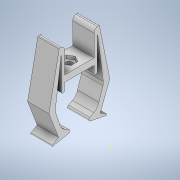
# Autodesk Inventor part: защёлка_выдача2
Saved by Autodesk Inventor 2020 (Build 240168000, 168)
## iProperties
Created: 2022-07-29
Part Number: защёлка_выдача2
Material: Типовые
Document SubType Name: Modeling
Designer: akapu
Density: 1 g/cm^3
Appearance: По умолчанию
Author: akapu
Autodesk Inventor part; units mm, degrees
ref_plane "YZ Plane" through (0, 0, 0) normal (1, 0, 0) x (0, 1, 0)
ref_plane "XZ Plane" through (0, 0, 0) normal (0, 1, 0) x (-1, 0, 0)
ref_plane "XY Plane" through (0, 0, 0) normal (0, 0, 1) x (1, 0, 0)
sketch "Эскиз8" plane through (0, 0, 0) normal (1, 0, 0) x (0, 1, 0)
  line L0 (0, 0) -> (10.4, 0)
  line L1 (10.4, 0) -> (10.4, -10.4)
  line L2 (10.4, -10.4) -> (0, -10.4)
  line L3 (0, -10.4) -> (0, 0)
  line L4 (5.2, 0) -> (5.2, 4)
  line L5 (5.2, -10.4) -> (5.2, -14.4)
  circle A0 centre (5.2, 4) radius 1.6
  circle A1 centre (5.2, -14.4) radius 1.6
  line L6 (5.2, 4) -> (7.9, 4)
  line L7 (7.9, 2.4412) -> (5.2, 0.8823)
  line L8 (5.2, 0.8823) -> (2.5, 2.4412)
  line L9 (2.5, 2.4412) -> (2.5, 5.5588)
  line L10 (2.5, 5.5588) -> (5.2, 7.1177)
  line L11 (5.2, 7.1177) -> (7.9, 5.5588)
  line L12 (7.9, 5.5588) -> (7.9, 2.4412)
  line L13 (7.9, -15.9588) -> (5.2, -17.5177)
  line L14 (5.2, -17.5177) -> (2.5, -15.9588)
  line L15 (2.5, -15.9588) -> (2.5, -12.8412)
  line L16 (2.5, -12.8412) -> (5.2, -11.2823)
  line L17 (5.2, -11.2823) -> (7.9, -12.8412)
  line L18 (7.9, -12.8412) -> (7.9, -15.9588)
  circle A2 centre (5.2, 4) radius 5.2
  circle A3 centre (5.2, -14.4) radius 5.2
  line L19 (10.4, 4) -> (10.4, 0)
  line L20 (10.4, -10.4) -> (10.4, -14.4)
  line L21 (0, -14.4) -> (0, -10.4)
  line L22 (0, 4) -> (0, 0)
  line L23 (7.9, 5.5588) -> (7.9, 8.4441)
  line L24 (2.5, 5.5588) -> (2.5, 8.4441)
  line L25 (2.5, -15.9588) -> (2.5, -18.8441)
  line L26 (7.9, -15.9588) -> (7.9, -18.8441)
  line L27 (0, 0) -> (-3, 0)
  line L28 (-3, 0) -> (-3, -10.4)
  line L29 (-3, -10.4) -> (0, -10.4)
  line L30 (0, -10.4) -> (0, 0)
  line L31 (10.4, 0) -> (8.9, 2.5981)
  line L32 (10.4, -10.4) -> (8.9, -12.9981)
  line L33 (10.4, -10.4) -> (13.4, -10.4) construction
  line L34 (8.9, -12.9981) -> (4.4, -10.4)
  line L35 (8.9, 2.5981) -> (4.4, 0)
  line L36 (-3, 0) -> (0.663, 6.5408)
  line L37 (-3, -10.4) -> (0.663, -16.9408)
  line L38 (10.4, 0) -> (12.9981, 1.5)
  line L39 (12.9981, 1.5) -> (9.5707, 6.8173)
  line L40 (10.4, -10.4) -> (12.9981, -11.9)
  line L41 (12.9981, -11.9) -> (9.5707, -17.2173)
  point P0 (7.9, -14.4)
  dimension "d51" = 10.4
  dimension "d52" = 10.4
  dimension "d53" = 4
  dimension "d54" = 4
  dimension "d55" = 3.2
  dimension "d56" = 3.2
  dimension "d57" = 2.7
  dimension "d58" = 3
  dimension "d59" = 3
  dimension "d60" = 3
  dimension "d61" = 120
  dimension "d62" = 3
  dimension "d63" = 3
  constraints: 84 end point, 12 point on circle, 7 tangent, 6 coincident, 6 parallel, 6 point on line, 5 perpendicular, 4 centre point, 4 midpoint, 4 vertical, 3 horizontal, 1 collinear, 1 equal length, 26 other
  measures "d51" distance of L1.end L2.end
  measures "d52" distance of L0.end L1.end
  measures "d53" distance of L4.start L4.end
  measures "d54" distance of L5.start L5.end
  measures "d55" diameter of A0
  measures "d56" diameter of A1
  measures "d57" distance of L6.start L6.end
  measures "d58" distance of L29.end L28.end
  measures "d59" distance of L0.end L31.end
  measures "d60" distance of L1.end L32.end
  measures "d61" angle of L32 L33
  measures "d62" distance of L0.end L38.end
  measures "d63" distance of L1.end L40.end
extrude "Выдавливание6" add sketch "Эскиз8" along normal blind 5 contours L0 A2 L24 L9 L8 L4 L35 | L0 L22 A2 | L4 L7 L12 L23 A2 L31 L35 | L27 L36 A2 L22 | L3 L29 L28 L27 | L31 A2 L19 | L19 A2 L39 L38 | L2 A3 L21 | L21 A3 L37 L29 | L40 L41 A3 L20 | L20 A3 L32 | L2 L34 L5 L16 L15 L25 A3 | A3 L26 L18 L17 L5 L34 L32
sketch "Эскиз9" plane through (0, 0, 0) normal (-1, 0, 0) x (0, 0, 1)
  arc A0 (-18.8441, 2.5) -> (-16.9408, 0.663) centre (-14.4, 5.2) ccw projected
  circle A1 centre (-14.4, 5.2) radius 5.2
  circle A2 centre (-14.4, 5.2) radius 1.6
  arc A3 (6.5408, 0.663) -> (8.4441, 2.5) centre (4, 5.2) ccw projected
  circle A4 centre (4, 5.2) radius 5.2
  circle A5 centre (4, 5.2) radius 1.6
  line L0 (2.5981, 8.9) -> (0, 10.4) projected
  line L1 (0, 10.4) -> (2.5981, 8.9)
  line L2 (0, 4.4) -> (2.5981, 8.9) projected
  line L3 (2.5981, 8.9) -> (0, 4.4)
  line L4 (0, 0) -> (0, 4.4) projected
  line L5 (0, 4.4) -> (0, 0)
  line L6 (-10.4, 4.4) -> (-10.4, 0) projected
  line L7 (0, 0) -> (-10.4, 0)
  line L8 (-10.4, 0) -> (-10.4, 1.8774)
  line L9 (-10.4, 10.4) -> (-12.9981, 8.9) projected
  line L10 (-11.699, 9.65) -> (-10.4, 10.4)
  line L11 (-11.9, 12.9981) -> (-10.4, 10.4) projected
  line L12 (-10.4, 10.4) -> (-11.9, 12.9981)
  line L13 (-17.2173, 9.5707) -> (-11.9, 12.9981) projected
  line L14 (-11.9, 12.9981) -> (-17.2173, 9.5707)
  line L15 (0, 10.4) -> (1.5, 12.9981) projected
  line L16 (0, 10.4) -> (1.5, 12.9981)
  line L17 (1.5, 12.9981) -> (6.8173, 9.5707) projected
  line L18 (1.5, 12.9981) -> (6.8173, 9.5707)
  line L19 (0, -3) -> (-10.4, -3) projected
  line L20 (0, -3) -> (6.5408, 0.663)
  line L21 (6.5408, 0.663) -> (0, -3) projected
  line L22 (-10.4, -3) -> (-16.9408, 0.663)
  line L23 (-10.4, -3) -> (-16.9408, 0.663) projected
  line L24 (-10.4, -3) -> (0, -3)
  line L25 (-10.4, 0) -> (0, 0) projected
  line L26 (0, 0) -> (-10.4, 0)
  line L27 (-10.4, 0) -> (-10.4, 1.8774)
  line L28 (0, 1.8774) -> (0, 0)
  line L29 (-11.699, 9.65) -> (-12.9981, 8.9)
  line L30 (-12.9981, 8.9) -> (-10.4, 4.4) projected
  line L31 (-10.4, 4.4) -> (-12.9981, 8.9)
  line L32 (-12.9981, 8.9) -> (-10.4, 4.4)
  line L33 (-10.4, 4.4) -> (-10.4, 1.8774)
  line L34 (0, 1.8774) -> (0, 4.4)
  line L35 (2.5981, 8.9) -> (0, 4.4)
  line L36 (1.299, 9.65) -> (2.5981, 8.9)
  point P0 (-18.8441, 2.5)
  point P1 (-16.9408, 0.663)
  point P2 (6.5408, 0.663)
  point P3 (8.4441, 2.5)
  dimension "d66" = 3.2
  dimension "d67" = 3.2
  constraints: 46 end point, 14 collinear, 4 centre point, 4 coincident, 4 perpendicular, 4 point on circle, 3 point on line, 2 horizontal, 2 midpoint, 2 tangent, 1 parallel
  measures "d66" diameter of A2
  measures "d67" diameter of A5
extrude "Выдавливание7" add sketch "Эскиз9" along normal blind 5 contours A1 L9 L30 L6 A0 | A1 L6 L7 L4 A4 L20 L19 L22 | L13 L11 L9 A1 | A4 L4 L2 L0 A3 | L0 L15 L17 A4
sketch "Эскиз10" plane through (5, 0, 0) normal (1, 0, 0) x (0, 0, -1)
  line L0 (-1.5, 12.9981) -> (-6.8173, 9.5707) projected
  line L1 (0, 10.4) -> (-1.5, 12.9981) projected
  line L2 (-1.5, 12.9981) -> (0, 10.4)
  line L3 (-2.5981, 8.9) -> (0, 10.4) projected
  line L4 (0, 10.4) -> (-2.5981, 8.9)
  line L5 (0, 4.4) -> (-2.5981, 8.9) projected
  line L6 (-2.5981, 8.9) -> (0, 4.4)
  line L7 (0, 0) -> (0, 4.4) projected
  line L8 (0, 4.4) -> (0, 0)
  line L9 (10.4, 0) -> (0, 0) projected
  line L10 (0, 0) -> (10.4, 0)
  line L11 (10.4, 4.4) -> (10.4, 0) projected
  line L12 (10.4, 0) -> (10.4, 4.4)
  line L13 (10.4, 10.4) -> (12.9981, 8.9) projected
  line L14 (10.4, 4.4) -> (12.9981, 8.9)
  line L15 (12.9981, 8.9) -> (10.4, 10.4)
  line L16 (11.9, 12.9981) -> (10.4, 10.4) projected
  line L17 (10.4, 10.4) -> (11.9, 12.9981)
  line L18 (17.2173, 9.5707) -> (11.9, 12.9981) projected
  line L19 (11.9, 12.9981) -> (17.2173, 9.5707)
  line L20 (17.2173, 9.5707) -> (13.6704, -1.1685)
  line L21 (10.4, -3) -> (16.9408, 0.663) projected
  line L22 (10.4, -3) -> (13.6704, -1.1685)
  line L23 (0, -3) -> (10.4, -3) projected
  line L24 (-6.5408, 0.663) -> (0, -3) projected
  line L25 (10.4, -3) -> (0, -3)
  arc A0 (-8.4441, 2.5) -> (-6.5408, 0.663) centre (-4, 5.2) ccw projected
  line L26 (0, -3) -> (-6.5408, 0.663)
  line L27 (-3.2704, -1.1685) -> (-6.8173, 9.5707)
  line L28 (-6.8173, 9.5707) -> (-1.5, 12.9981)
  constraints: 32 end point, 9 collinear, 3 perpendicular, 2 midpoint, 1 tangent
extrude "Выдавливание8" add sketch "Эскиз10" along normal blind 157.53
sketch "Эскиз17" plane through (-5, 0, 0) normal (-1, 0, 0) x (0, 0, 1)
  line L0 (-37.7292, 41.1824) -> (41.3103, 41.1824)
  line L1 (41.3103, 41.1824) -> (41.3103, -34.7876)
  line L2 (41.3103, -34.7876) -> (-37.7292, -34.7876)
  line L3 (-37.7292, -34.7876) -> (-37.7292, 41.1824)
  point P0 (0, 0)
  constraints: 8 end point, 2 parallel, 1 horizontal, 1 perpendicular
extrude "Выдавливание13" cut sketch "Эскиз17" against normal blind 147.53
sketch "Эскиз23" plane through (162.53, 0, 0) normal (1, 0, 0) x (0, 0, -1)
  point P0 (0, 0)
fillet "Сопряжение12" radius 4 6 edges at (152.53, -3, -10.4) (152.53, -1.1685, -13.6704) (152.53, -3, 0) (152.53, -1.1685, 3.2704) (152.53, 9.5707, -17.2173) (152.53, 9.5707, 6.8173)
sketch "Эскиз24" plane through (142.53, 0, 0) normal (-1, 0, 0) x (0, 0, 1)
  line L0 (-11.9, 12.9981) -> (-10.4, 10.4) projected
  line L1 (-11.9, 12.9981) -> (1.5, 12.9981)
  line L2 (1.5, 12.9981) -> (1.5, 16.9981)
  line L3 (1.5, 16.9981) -> (-11.9, 16.9981)
  line L4 (-11.9, 16.9981) -> (-11.9, 12.9981)
  line L5 (1.5, 16.9981) -> (-11.9, 16.9981)
  line L6 (-11.9, 16.9981) -> (-11.9, 19.9981)
  line L7 (-11.9, 19.9981) -> (1.5, 19.9981)
  line L8 (1.5, 19.9981) -> (1.5, 16.9981)
  line L9 (-11.9, 16.9981) -> (-11.7, 16.9981) construction
  line L10 (-14.6154, 11.2478) -> (-11.9, 12.9981) projected
  line L11 (-12.1, 12.9981) -> (-11.9, 12.9981)
  line L12 (1.5, 12.9981) -> (1.7, 12.9981)
  line L13 (1.7, 13.7481) -> (1.7, 19.9981)
  line L14 (1.7, 19.9981) -> (1.5, 19.9981)
  line L15 (-12.1, 13.7481) -> (-12.1, 19.9981)
  line L16 (-12.1, 19.9981) -> (-11.9, 19.9981)
  line L17 (-12.1, 16.9981) -> (-11.9, 16.9981)
  line L18 (1.5, 16.9981) -> (1.7, 16.9981)
  line L19 (-12.85, 12.9981) -> (-12.85, 12.9981)
  line L20 (-13.6, 13.7481) -> (-13.6, 28.4571)
  line L21 (-13.6, 29.9981) -> (-12.1, 29.9981)
  line L22 (-12.1, 29.9981) -> (-12.1, 12.9981)
  line L23 (2.45, 12.9981) -> (2.45, 12.9981)
  line L24 (3.2, 13.7481) -> (3.2, 28.4571)
  line L25 (3.2, 29.9981) -> (1.7, 29.9981)
  line L26 (1.7, 29.9981) -> (1.7, 12.9981)
  line L27 (-13.7992, 28.47) -> (-16.4147, 8.4027)
  arc A0 (-14.6154, 11.2478) -> (-16.2465, 6.6313) centre (-12.4482, 7.8857) ccw projected
  line L28 (3.3992, 28.47) -> (6.0147, 8.4027)
  arc A1 (5.8465, 6.6313) -> (4.2154, 11.2478) centre (2.0482, 7.8857) ccw projected
  arc A2 (-12.85, 12.9981) -> (-12.1, 13.7481) centre (-12.85, 13.7481) ccw
  arc A3 (-13.6, 13.7481) -> (-12.85, 12.9981) centre (-12.85, 13.7481) ccw
  arc A4 (1.7, 13.7481) -> (2.45, 12.9981) centre (2.45, 13.7481) ccw
  arc A5 (2.45, 12.9981) -> (3.2, 13.7481) centre (2.45, 13.7481) ccw
  line L29 (-14.1579, 0.3075) -> (-16.2465, 6.6313) projected
  line L30 (-16.2465, 6.6313) -> (-14.1579, 0.3075)
  circle A6 centre (-12.4482, 7.8857) radius 4
  line L31 (5.8465, 6.6313) -> (3.7579, 0.3075) projected
  circle A7 centre (2.0482, 7.8857) radius 4
  arc A8 (1.9142, -1.928) -> (3.7579, 0.3075) centre (-0.0403, 1.562) ccw projected
  circle A9 centre (-0.0403, 1.562) radius 4
  arc A10 (-1.0438, -3) -> (0.9107, -2.49) centre (-1.0438, 1) ccw projected
  circle A11 centre (-1.0438, 1) radius 4
  line L32 (-10.4, 4.4) -> (-10.4, 0) projected
  circle A12 centre (-10.4, 1.562) radius 4.0051
  arc A13 (-11.3107, -2.49) -> (-9.3562, -3) centre (-9.3562, 1) ccw projected
  circle A14 centre (-9.3562, 1) radius 4
  arc A15 (-14.1579, 0.3075) -> (-12.3142, -1.928) centre (-10.3597, 1.562) ccw projected
  line L33 (-12.3142, -1.928) -> (-11.3107, -2.49)
  line L34 (1.9142, -1.928) -> (0.9107, -2.49) projected
  line L35 (1.9142, -1.928) -> (0.9107, -2.49)
  line L36 (-1.0438, -3) -> (-9.3562, -3) projected
  line L37 (-9.3562, -3) -> (-1.0438, -3)
  line L38 (0.9107, -2.49) -> (-0.2774, -3.1554)
  line L39 (-11.3107, -2.49) -> (-10.1226, -3.1554)
  line L40 (2.0482, 7.8857) -> (6.0482, 7.8857)
  line L41 (6.0482, 7.8857) -> (9.0482, 7.8857)
  line L42 (-16.4482, 7.8857) -> (-19.4482, 7.8857)
  line L43 (-19.4482, 7.8857) -> (-14.9537, -3.9206)
  line L44 (-13.6, 29.9981) -> (-13.6, 31.9981)
  line L45 (3.2, 29.9981) -> (3.2, 31.9981)
  arc A16 (3.2, 31.9981) -> (1.7, 29.9981) centre (3.699, 30.0613) ccw
  arc A17 (-12.1, 29.9981) -> (-13.6, 31.9981) centre (-14.099, 30.0613) ccw
  arc A18 (3.3992, 28.47) -> (3.2, 28.4571) centre (3.3, 28.4571) ccw
  arc A19 (-13.6, 28.4571) -> (-13.7992, 28.47) centre (-13.7, 28.4571) ccw
  line L46 (3.2, 31.9981) -> (4.2, 31.9976)
  line L47 (4.2, 31.9976) -> (9.0482, 7.8857)
  line L48 (-13.6, 31.9981) -> (-14.6, 31.9981)
  line L49 (-14.6, 31.9981) -> (-19.4482, 7.8857)
  line L50 (9.0482, 7.8857) -> (4.5537, -3.9206)
  circle A20 centre (0.1512, -3.9206) radius 0.8771
  circle A21 centre (-10.5512, -3.9206) radius 0.8771
  line L51 (4.5537, -3.9206) -> (9.0482, -6.5155)
  line L52 (4.5537, -3.9206) -> (9.7436, -3.9206) construction
  line L53 (9.0482, -6.5155) -> (-0.0136, -4.7821)
  line L54 (-14.9537, -3.9206) -> (-19.4482, -6.5155)
  line L55 (-14.9537, -3.9206) -> (-9.7638, -3.9206) construction
  line L56 (-19.4482, -6.5155) -> (-10.3864, -4.7821)
  point P0 (0, 0)
  point P1 (-13.6, 12.9981)
  point P2 (3.2, 12.9981)
  point P3 (-15.1183, -5.3024)
  point P4 (-11.3107, -2.49)
  point P5 (-11.9564, -2.1284)
  point P6 (-14.3463, 0.8779)
  dimension "d145" = 4
  dimension "d149" = 0.2
  dimension "d150" = 1.5
  dimension "d151" = 17
  dimension "d152" = 1.5
  dimension "d153" = 17
  dimension "d154" = 0.75
  dimension "d161" = 3
  dimension "d162" = 3
  dimension "d163" = 2
  dimension "d164" = 2
  dimension "d165" = 2
  dimension "d166" = 0.1
  dimension "d167" = 1
  dimension "d168" = 1
  dimension "d187" = 30
  dimension "d188" = 150
  constraints: 100 end point, 29 point on circle, 22 tangent, 19 point on line, 14 centre point, 12 horizontal, 9 parallel, 9 perpendicular, 5 coincident, 4 collinear, 4 equal radius, 2 equal length, 1 vertical, 1 vertical alignment, 8 other
  measures "d145" distance of L2.end L1.end
  measures "d149" distance of L1.end L12.end
  measures "d150" distance of L21.start L21.end
  measures "d151" distance of point (-13.6, 12.998) L21.start
  measures "d152" distance of L25.end L25.start
  measures "d153" distance of L25.start point (3.2, 12.998)
  measures "d154" radius of A2
  measures "d161" distance of L40.end L41.end
  measures "d162" distance of L42.start L42.end
  measures "d163" distance of L21.start L44.end
  measures "d164" radius of A16
  measures "d165" radius of A17
  measures "d166" radius of A18
  measures "d167" distance of L45.end L46.end
  measures "d168" distance of L44.end L48.end
  measures "d187" angle of L51 L52
  measures "d188" angle of L54 L55
extrude "Выдавливание17" add sketch "Эскиз24" along normal blind 10 contours L6 L7 L8 L3 | L17 L15 L16 L6 | L8 L14 L13 L18 | L15 A2 A3 L20 A19 L27 A0 L42 L49 L48 L44 L21 L22 | L13 L26 L25 L45 L46 L47 L41 A1 L28 A18 L24 A5 A4 | A0 L29 A12 L33 L39 A21 L56 L54 L43 L42 | L21 L44 A17 | A16 L45 L25 | A21 | L34 A8 L31 A1 L41 L50 L51 L53 A20 L38 | A20
fillet "Сопряжение13" radius 0.3 4 edges at (137.53, 31.9976, 4.2) (137.53, 31.9981, -14.6) (137.53, -6.5155, 9.0482) (137.53, -6.5155, -19.4482)
sketch "Эскиз25" plane through (162.53, 0, 0) normal (1, 0, 0) x (0, 0, -1)
  line L0 (-19.4307, 22.3831) -> (30.691, 22.3831)
  line L1 (30.691, 22.3831) -> (30.691, -15.6545)
  line L2 (30.691, -15.6545) -> (-19.4307, -15.6545)
  line L3 (-19.4307, -15.6545) -> (-19.4307, 22.3831)
  point P0 (0, 0)
  constraints: 8 end point, 2 parallel, 1 horizontal, 1 perpendicular
extrude "Выдавливание18" cut sketch "Эскиз25" against normal blind 20
sketch "Эскиз28" plane through (132.53, 19.9981, -12.1) normal (0, 1, 0) x (1, 0, 0)
  line L0 (0, -13.8) -> (0, 0) projected
  line L1 (0, -6.9) -> (10, -6.9)
  line L2 (10, -13.8) -> (10, 0) projected
  circle A0 centre (5, -6.9) radius 1.6
  point P0 (-132.53, -12.1)
  dimension "d189" = 3.2
  constraints: 3 midpoint, 2 end point, 1 centre point
  measures "d189" diameter of A0
extrude "Выдавливание21" cut sketch "Эскиз28" against normal blind 10
sketch "Эскиз29" plane through (132.53, 19.9981, -12.1) normal (0, 1, 0) x (1, 0, 0)
  circle A0 centre (5, -6.9) radius 1.6 projected
  line L0 (5, -6.9) -> (7.7, -6.9)
  line L1 (7.7, -8.4588) -> (5, -10.0177)
  line L2 (5, -10.0177) -> (2.3, -8.4588)
  line L3 (2.3, -8.4588) -> (2.3, -5.3412)
  line L4 (2.3, -5.3412) -> (5, -3.7823)
  line L5 (5, -3.7823) -> (7.7, -5.3412)
  line L6 (7.7, -5.3412) -> (7.7, -8.4588)
  point P0 (-132.53, -12.1)
  dimension "d192" = 2.7
  constraints: 14 end point, 1 coincident, 1 horizontal, 1 midpoint, 13 other
  measures "d192" distance of L0.start L0.end
extrude "Выдавливание22" cut sketch "Эскиз29" against normal blind 1.5
